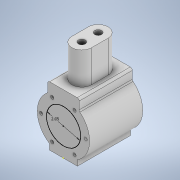
# Autodesk Inventor part: examen
Saved by Autodesk Inventor 2020 (Build 240168000, 168)
## iProperties
Created: 2020-03-09
Part Number: examen
Material: Genérico
Document SubType Name: Modeling
Designer: luisg
Density: 1 g/cm^3
Appearance: Valor por defecto
Author: luisg
Autodesk Inventor part; units mm, degrees
ref_plane "YZ Plane" through (0, 0, 0) normal (1, 0, 0) x (0, 1, 0)
ref_plane "XZ Plane" through (0, 0, 0) normal (0, 1, 0) x (-1, 0, 0)
ref_plane "XY Plane" through (0, 0, 0) normal (0, 0, 1) x (1, 0, 0)
sketch "Boceto1" plane through (0, 0, 0) normal (0, 0, 1) x (1, 0, 0)
  circle A0 centre (0, 0) radius 1.57
  line L0 (0, 0) -> (1.34, 0) construction
  line L1 (0, 0) -> (-1.34, 0) construction
  circle A1 centre (-1.34, 0) radius 0.095
  circle A2 centre (-0.67, 1.1605) radius 0.095
  circle A3 centre (0, 0) radius 1.57
  circle A4 centre (0.67, 1.1605) radius 0.095
  circle A5 centre (0, 0) radius 1.57
  circle A6 centre (1.34, 0) radius 0.095
  circle A7 centre (0, 0) radius 1.57
  circle A8 centre (0.67, -1.1605) radius 0.095
  circle A9 centre (0, 0) radius 1.57
  circle A10 centre (-0.67, -1.1605) radius 0.095
  circle A11 centre (0, 0) radius 1.57
  line L2 (-0.67, 1.1605) -> (0.67, 1.1605) construction
  line L3 (0, 0) -> (-0.67, 1.1605) construction
  circle A12 centre (0, 0) radius 1.17
  line L4 (-0.945, 1.2537) -> (-0.945, 1.89)
  line L5 (-0.945, 1.89) -> (0.945, 1.89)
  line L6 (0.945, 1.89) -> (0.945, 1.2537)
  line L7 (0, 2.3163) -> (0, 0) construction
  line L8 (0.84, -1.3264) -> (0.84, -1.6664)
  line L9 (0.84, -1.6664) -> (-0.84, -1.6664)
  line L10 (-0.84, -1.6664) -> (-0.84, -1.3264)
  point P0 (0, 1.89)
  dimension "d0" = 3.14
  dimension "d4" = 0.19
  dimension "d7" = 360
  dimension "d9" = 1.34
  dimension "d10" = 1.34
  dimension "d11" = 2.34
  dimension "d12" = 1.89
  dimension "d13" = 1.89
  dimension "d34" = 0.34
  dimension "d35" = 0.34
  dimension "d36" = 0.84
  constraints: 22 end point, 13 centre point, 5 coincident, 5 perpendicular, 4 point on circle, 3 horizontal, 3 point on line, 2 vertical, 1 midpoint, 23 other
  measures "d0" diameter of A0
  measures "d4" diameter of A1
  measures "d9" distance of L2.start L2.end
  measures "d10" distance of L2.start point (0, 0)
  measures "d11" diameter of A12
  measures "d12" distance between parallel lines of L4 L6
  measures "d13" distance between parallel lines of L1 L5
  measures "d34" distance of L8.start L8.end
  measures "d35" distance of L9.end L10.end
  measures "d36" distance between parallel lines of L8 L7
extrude "Extrusión1" add sketch "Boceto1" against normal blind 3.19 contours A0 | A0 L4 L5 L6 | L8 L9 L10 A0 | A12
fillet "Empalme1" radius 0.12 4 edges at (0.945, 1.2537, -1.595) (0.945, 1.89, -1.595) (-0.945, 1.2537, -1.595) (-0.945, 1.89, -1.595)
sketch "Boceto2" plane through (-0.825, 1.89, 0) normal (0, 1, 0) x (1, 0, 0)
  line L0 (0, 0) -> (0, 3.19) construction
  line L1 (1.65, 0) -> (0, 0) construction
  line L2 (1.65, 3.19) -> (1.65, 0) construction
  line L3 (0, 3.19) -> (1.65, 3.19) construction
  line L4 (0.06, 3.19) -> (0.06, 0) construction
  line L5 (0.06, 1.595) -> (1.65, 1.595) construction
  line L6 (1.65, 3.19) -> (1.65, 0) construction
  line L7 (0.825, 2.68) -> (0.825, 0.51) construction
  line L8 (0.825, 0) -> (0.825, 3.1487) construction
  line L9 (-0.015, 3.19) -> (-0.745, 3.19) construction
  line L10 (0.235, 2.09) -> (0.235, 1.1)
  line L11 (1.415, 2.09) -> (1.415, 1.1)
  circle A0 centre (0.825, 2.085) radius 0.21
  circle A1 centre (0.825, 1.105) radius 0.21
  arc A2 (1.415, 2.09) -> (0.235, 2.09) centre (0.825, 2.09) ccw
  arc A3 (0.235, 1.1) -> (1.415, 1.1) centre (0.825, 1.1) ccw
  point P0 (1.8144, 3.19)
  point P1 (-0.1644, 3.19)
  point P2 (0.825, 1.595)
  point P3 (0.825, 1.5744)
  point P4 (0.5472, 0.7661)
  dimension "d17" = 2.17
  dimension "d18" = 1.085
  dimension "d22" = 0.42
  dimension "d23" = 0.42
  dimension "d24" = 0.98
  dimension "d25" = 0.49
  dimension "d26" = 0.59
  dimension "d27" = 0.59
  dimension "d38" = 180
  constraints: 10 end point, 6 point on circle, 6 point on line, 4 centre point, 3 midpoint, 2 tangent, 1 parallel, 1 perpendicular, 1 vertical
  measures "d17" distance of L7.start L7.end
  measures "d18" distance from line of L5 L7.start
  measures "d22" diameter of A0
  measures "d23" diameter of A1
  measures "d24" distance of A1.centre A0.centre
  measures "d25" distance from line of L5 A0.centre
  measures "d26" radius of A2
  measures "d27" radius of A3
  measures "d38" angle of L8 L7
extrude "Extrusión2" add sketch "Boceto2" along normal blind 1.93
sketch "Boceto3" plane through (0, 0, 0) normal (0, 0, 1) x (1, 0, 0)
  circle A0 centre (0, 0) radius 1.025
  dimension "d31" = 2.05
  constraints: 1 centre point, 1 coincident
  measures "d31" diameter of A0
sketch "Boceto7" plane through (-0.84, -1.6664, 0) normal (0, -1, 0) x (1, 0, 0)
  point P0 (0.84, 0)
